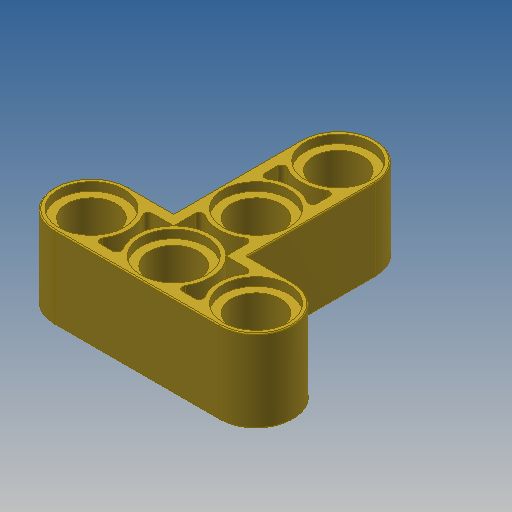
# Autodesk Inventor part: 60484-Yellow
Saved by Autodesk Inventor 2022.2 (Build 262287000, 287)
## iProperties
Created: 2012-03-21
Part Number: 60484-Yellow
Document SubType Name: Modeling
Designer: D. Kohfeld
Density: 1.06 g/cm^3
Material: ABS Plastic
Mass: 1.19791 g
Surface Area: 20.1744 cm^2
Volume: 1.13011 cm^3
Appearance: Yellow
Author: D. Kohfeld
Autodesk Inventor part; units mm, degrees
ref_plane "YZ Plane" through (0, 0, 0) normal (1, 0, 0) x (0, 1, 0)
ref_plane "XZ Plane" through (0, 0, 0) normal (0, 1, 0) x (-1, 0, 0)
ref_plane "XY Plane" through (0, 0, 0) normal (0, 0, 1) x (1, 0, 0)
sketch "Sketch1" plane through (0, 0, 0) normal (0, 0, 1) x (1, 0, 0)
  line L0 (3.6, -4.4) -> (3.6, 8)
  line L1 (-3.6, 8) -> (-3.6, -4.4)
  arc A0 (3.6, 8) -> (-3.6, 8) centre (0, 8) ccw
  circle A1 centre (0, 8) radius 2.4
  circle A2 centre (0, 8) radius 3.2
  circle A3 centre (0, 0) radius 3.2
  circle A4 centre (0, 0) radius 2.4
  line L2 (0, 0) -> (0, 8) construction
  line L3 (-2.5456, 5.4544) -> (-2.5456, 2.5456)
  line L4 (2.5456, 5.4544) -> (2.5456, 2.5456)
  arc A5 (-2.5456, 5.4544) -> (2.5456, 5.4544) centre (0, 8) ccw
  arc A6 (2.5456, 2.5456) -> (-2.5456, 2.5456) centre (0, 0) ccw
  arc A7 (-3.6, -8) -> (3.6, -8) centre (0, -8) ccw construction
  circle A8 centre (0, -8) radius 3.2
  circle A9 centre (0, -8) radius 2.4
  line L5 (0, 0) -> (0, -8) construction
  line L6 (-2.5456, -2.5456) -> (-2.5456, -5.4544)
  line L7 (2.5456, -2.5456) -> (2.5456, -5.4544)
  arc A10 (-2.5456, -2.5456) -> (2.5456, -2.5456) centre (0, 0) ccw
  arc A11 (2.5456, -5.4544) -> (-2.5456, -5.4544) centre (0, -8) ccw
  line L8 (0, -8) -> (-2.5456, -5.4544) construction
  line L9 (-8, -11.6) -> (8, -11.6)
  arc A12 (8, -11.6) -> (8, -4.4) centre (8, -8) ccw
  line L10 (8, -4.4) -> (3.6, -4.4)
  arc A13 (-8, -4.4) -> (-8, -11.6) centre (-8, -8) ccw
  line L11 (-8, -4.4) -> (-3.6, -4.4)
  circle A14 centre (-8, -8) radius 3.2
  circle A15 centre (-8, -8) radius 2.4
  circle A16 centre (8, -8) radius 3.2
  circle A17 centre (8, -8) radius 2.4
  line L12 (-8, -8) -> (0, -8) construction
  line L13 (8, -8) -> (0, -8) construction
  dimension "d8" = 4.8
  dimension "d9" = 6.4
  dimension "d32" = 7.2
  dimension "d34" = 8
  dimension "d47" = 45
  constraints: 28 end point, 18 centre point, 16 point on circle, 14 coincident, 14 equal radius, 9 tangent, 6 equal length, 6 parallel, 3 perpendicular, 2 vertical, 1 collinear
  measures "d8" diameter of A1
  measures "d9" diameter of A2
  measures "d32" diameter of A0
  measures "d34" distance of L2.start L2.end
  measures "d47" angle of L5 L8
extrude "Extrusion1" add sketch "Sketch1" along normal mid plane 8 contours L10 A12 L9 A13 L11 L1 A0 L0 | A2 | A3 | A5 L4 A6 L3 | A8 | A10 L7 A11 L6 | A14 | A16
sketch "Sketch6" plane through (0, 0, 4) normal (0, 0, 1) x (1, 0, 0)
  circle A0 centre (0, 0) radius 2.4 projected
  circle A1 centre (0, 8) radius 2.4 projected
  circle A2 centre (0, 0) radius 3.2 projected
  circle A3 centre (0, 8) radius 3.2 projected
  arc A4 (2.5456, 2.5456) -> (-2.5456, 2.5456) centre (0, 0) ccw projected
  line L0 (-2.5456, 5.4544) -> (-2.5456, 2.5456) projected
  arc A5 (-2.5456, 5.4544) -> (2.5456, 5.4544) centre (0, 8) ccw projected
  line L1 (2.5456, 5.4544) -> (2.5456, 2.5456) projected
  line L2 (-2.5456, -2.5456) -> (-2.5456, -5.4544) projected
  arc A6 (-2.5456, -2.5456) -> (2.5456, -2.5456) centre (0, 0) ccw projected
  arc A7 (2.5456, -5.4544) -> (-2.5456, -5.4544) centre (0, -8) ccw projected
  line L3 (2.5456, -2.5456) -> (2.5456, -5.4544) projected
  circle A8 centre (0, -8) radius 3.2 projected
  circle A9 centre (0, -8) radius 2.4 projected
  circle A10 centre (8, -8) radius 2.4 projected
  circle A11 centre (-8, -8) radius 2.4 projected
  line L4 (3.6, 8) -> (3.6, -4.4) projected
  line L5 (-2.5456, -5.4544) -> (-5.4544, -5.4544)
  line L6 (-2.5456, -10.5456) -> (-5.4544, -10.5456)
  line L7 (2.5456, -5.4544) -> (5.4544, -5.4544)
  line L8 (5.4544, -10.5456) -> (2.5456, -10.5456)
  arc A12 (-2.5456, -5.4544) -> (-2.5456, -10.5456) centre (0, -8) ccw
  arc A13 (-5.4544, -10.5456) -> (-5.4544, -5.4544) centre (-8, -8) ccw
  arc A14 (2.5456, -10.5456) -> (2.5456, -5.4544) centre (0, -8) ccw
  arc A15 (5.4544, -5.4544) -> (5.4544, -10.5456) centre (8, -8) ccw
  arc A16 (-8, -4.4) -> (-8, -11.6) centre (-8, -8) ccw projected
  arc A17 (8, -11.6) -> (8, -4.4) centre (8, -8) ccw projected
  circle A18 centre (-8, -8) radius 3.2
  circle A19 centre (8, -8) radius 3.2
  constraints: 8 end point, 8 point on circle, 6 centre point, 6 equal radius, 4 concentric, 4 parallel, 2 coincident, 1 perpendicular
extrude "Extrusion7" cut sketch "Sketch6" against normal blind 0.8 contours A2 | A3 | A8 | A18 | A19
extrude "Extrusion8" cut sketch "Sketch6" against normal blind 3.1 contours A4 L0 A5 L1 | A6 L3 A7 L2 | L7 A15 L8 A14 | A12 L6 A13 L5
mirror "Mirror1" about plane through (0, 0, 0) normal (0, 0, 1) of "Extrusion7", "Extrusion8"
fillet "Fillet1" radius 0.1 16 edges at (0, 11.6, 4) (3.6, 1.8, 4) (-3.6, 1.8, 4) (0, 11.6, -4) (-3.6, 1.8, -4) (3.6, 1.8, -4) (0, -11.6, 4) (-11.6, -8, 4) (-5.8, -4.4, 4) (5.8, -4.4, 4) (11.6, -8, 4) (5.8, -4.4, -4) (0, -11.6, -4) (-11.6, -8, -4) (-5.8, -4.4, -4) (11.6, -8, -4)
fillet "Fillet1" radius 0.4 24 edges at (-2.5456, 5.4544, 2.45) (-2.5456, 2.5456, 2.45) (2.5456, 2.5456, 2.45) (2.5456, 5.4544, 2.45) (2.5456, -2.5456, 2.45) (5.4544, -5.4544, 2.45) (5.4544, -10.5456, 2.45) (2.5456, -10.5456, 2.45) (-2.5456, -10.5456, 2.45) (-5.4544, -10.5456, 2.45) (-5.4544, -5.4544, 2.45) (-2.5456, -2.5456, 2.45) (-2.5456, 2.5456, -2.45) (-2.5456, 5.4544, -2.45) (2.5456, 5.4544, -2.45) (2.5456, 2.5456, -2.45) (-2.5456, -2.5456, -2.45) (2.5456, -2.5456, -2.45) (5.4544, -5.4544, -2.45) (5.4544, -10.5456, -2.45) (2.5456, -10.5456, -2.45) (-5.4544, -5.4544, -2.45) (-5.4544, -10.5456, -2.45) (-2.5456, -10.5456, -2.45)
equation "\"d8\" = tpd"
equation "\"d9\" = tsd"
equation "\"d32\" = tlad"
equation "\"d34\" = lu"
equation "\"d14\" = lu"
equation "\"d41\" = tsl"
equation "\"d45\" = lf"
equation "\"d48\" = tf"
equation "\"tpd\" = 4.8"
equation "\"tsd\" = 6.4"
equation "\"tlad\" = 7.2"
equation "\"lu\" = 8"
equation "\"tsl\" = 0.8"
equation "\"lf\" = 0.1"
equation "\"tf\" = 0.4"
body "Solid1"
